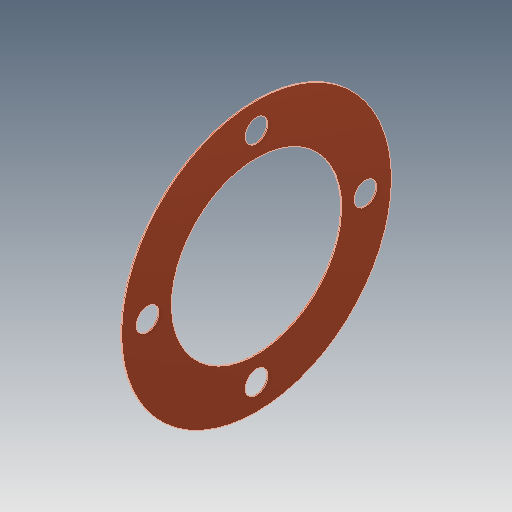
# Autodesk Inventor part: 低速轴承调整垫片
Saved by Autodesk Inventor 2025 (Build 290162000, 162)
## iProperties
Created: 2025-03-14
Part Number: 低速轴承调整垫片
Material: 铜，锻铸
Document SubType Name: Modeling
Designer: ASUS
Density: 8.94 g/cm^3
Appearance: 铜 - 缎光
Author: ASUS
Autodesk Inventor part; units mm, degrees
ref_plane "YZ Plane" through (0, 0, 0) normal (1, 0, 0) x (0, 1, 0)
ref_plane "XZ Plane" through (0, 0, 0) normal (0, 1, 0) x (-1, 0, 0)
ref_plane "XY Plane" through (0, 0, 0) normal (0, 0, 1) x (1, 0, 0)
sketch "草图1" plane through (0, 0, 0) normal (1, 0, 0) x (0, 1, 0)
  circle A0 centre (0, 0) radius 65
  circle A1 centre (0, 0) radius 41
  circle A2 centre (52.5, 0) radius 5.5
  circle A3 centre (0, 52.5) radius 5.5
  circle A4 centre (-52.5, 0) radius 5.5
  circle A5 centre (0, -52.5) radius 5.5
  dimension "d1" = 130
  dimension "d3" = 82
  dimension "d4" = 11
  dimension "d5" = 52.5
  dimension "d8" = 360
  constraints: 6 centre point, 2 coincident, 9 other
  measures "d1" diameter of A0
  measures "d3" diameter of A1
  measures "d4" diameter of A2
  measures "d5" distance of point (0, 0) A2.centre
extrude "拉伸1" add sketch "草图1" along normal blind 0.5
equation "\"d1\" = D2"
equation "\"d3\" = d2"
equation "\"d4\" = d0"
equation "\"d5\" = 0.5 * D0"
equation "\"d10\" = b"
equation "\"b\" = 0.5"
equation "\"d0\" = 11"
equation "\"D0\" = 105"
equation "\"d2\" = 82"
equation "\"D2\" = 130"
